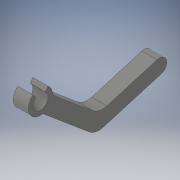
# Autodesk Inventor part: Holder left arm
Saved by Autodesk Inventor 2019.2 (Build 232265000, 265)
## iProperties
Created: 2020-09-20
Part Number: Holder left arm
Material: Generic
Document SubType Name: Modeling
Designer: SnoBotics
Density: 1 g/cm^3
Appearance: Rubber - Black(1)
Author: SnoBotics
Autodesk Inventor part; units mm, degrees
ref_plane "YZ Plane" through (0, 0, 0) normal (1, 0, 0) x (0, 1, 0)
ref_plane "XZ Plane" through (0, 0, 0) normal (0, 1, 0) x (-1, 0, 0)
ref_plane "XY Plane" through (0, 0, 0) normal (0, 0, 1) x (1, 0, 0)
sketch "Sketch1" plane through (0, 0, 0) normal (0, 0, 1) x (1, 0, 0)
  line L0 (7.0984, -37.2544) -> (-17.2546, -44.4717)
  line L1 (-19.0349, -38.4646) -> (5.3181, -31.2472)
  arc A0 (7.0984, -37.2544) -> (5.3181, -31.2472) centre (6.2488, -34.2388) ccw
  line L2 (-42.5288, -26.9478) -> (-20.5002, -45.4336)
  line L3 (-20.5002, -45.4336) -> (-17.2546, -44.4717)
  line L4 (-38.4744, -22.1514) -> (-19.0349, -38.4646)
  line L5 (-40.3781, -18.0047) -> (-41.5692, -19.4938)
  line L6 (-45.5333, -19.4938) -> (-46.7244, -18.0047)
  arc A1 (-45.5333, -19.4938) -> (-41.5692, -19.4938) centre (-43.5513, -21.9717) ccw
  arc A2 (-46.7244, -18.0047) -> (-42.5288, -26.9478) centre (-43.5513, -21.9717) ccw
  arc A3 (-38.4744, -22.1514) -> (-40.3781, -18.0047) centre (-43.5513, -21.9717) ccw
  point P0 (0, 0)
  point P1 (0, 0)
  constraints: 14 end point, 8 point on circle, 4 centre point, 2 concentric, 1 collinear, 1 parallel
extrude "Extrusion1" add sketch "Sketch1" along normal blind 6.35
fillet "Fillet1" radius 6.35 2 edges at (-20.5002, -45.4336, 3.175) (-19.0349, -38.4646, 3.175)
body "Solid1"
